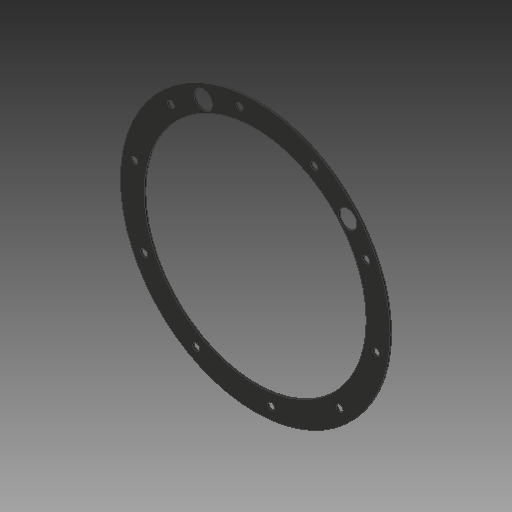
# Autodesk Inventor part: 1138_Inner Gasket_V1
Saved by Autodesk Inventor 2020 (Build 240168000, 168)
## iProperties
Created: 2019-05-13
Part Number: 1138_Inner Gasket_V1
Material: Rubber
Document SubType Name: Modeling
Designer: e22ma
Density: 0.93 g/cm^3
Appearance: Rubber - Black
Author: e22ma
Autodesk Inventor part; units mm, degrees
ref_plane "YZ Plane" through (0, 0, 0) normal (1, 0, 0) x (0, 1, 0)
ref_plane "XZ Plane" through (0, 0, 0) normal (0, 1, 0) x (-1, 0, 0)
ref_plane "XY Plane" through (0, 0, 0) normal (0, 0, 1) x (1, 0, 0)
sketch "Sketch1" plane through (0, 0, 0) normal (0, 0, 1) x (1, 0, 0)
  circle A0 centre (127.1655, 27.2155) radius 1.8415 projected
  circle A1 centre (12.2805, -27.2155) radius 1.8415 projected
  circle A2 centre (61.5903, 63.0411) radius 1.8415 projected
  circle A3 centre (7.2542, 11.7461) radius 1.8415 projected
  circle A4 centre (132.1918, -11.7461) radius 1.8415 projected
  circle A5 centre (100.1981, 55.7816) radius 1.8415 projected
  circle A6 centre (39.2479, -55.7816) radius 1.8415 projected
  circle A7 centre (77.8557, -63.0411) radius 1.8415 projected
  circle A8 centre (26.0889, 46.221) radius 1.8415 projected
  circle A9 centre (113.3571, -46.221) radius 1.8415 projected
  circle A10 centre (42.8005, 56.7029) radius 4.7625 projected
  circle A11 centre (117.5257, 40.681) radius 4.7625 projected
  circle A12 centre (69.723, 0) radius 57.404 projected
  circle A13 centre (69.723, 0) radius 69.723 projected
  point P0 (0, 0)
  constraints: 1 horizontal alignment
extrude "Extrusion1" add sketch "Sketch1" along normal blind 0.7937
body "Solid1"
